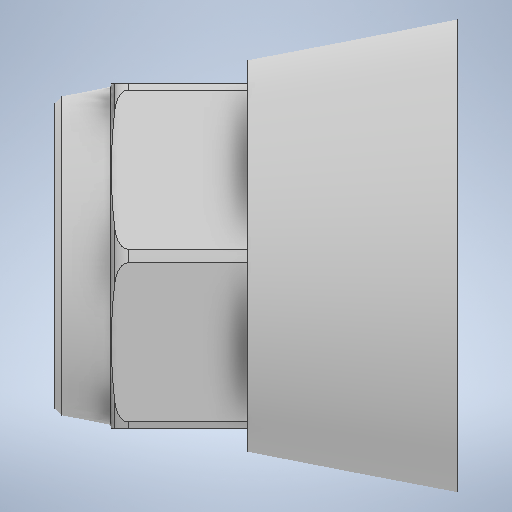
# Autodesk Inventor part: DT-HEX DWG_20251124
Saved by Autodesk Inventor 2025.3 (Build 293356000, 356)
## iProperties
Created: 2022-05-07
Part Number: DT-HEX DWG_20251124
Material: 일반
Document SubType Name: Modeling
Designer: shlee
Mass: 0.00932573 g
Surface Area: 0.529254 cm^2
Volume: 0.00932573 cm^3
Density: 1 g/cm^3
Appearance: 기본값
Author: shlee
Autodesk Inventor part; units mm, degrees
ref_plane "YZ Plane" through (0, 0, 0) normal (1, 0, 0) x (0, 1, 0)
ref_plane "XZ Plane" through (0, 0, 0) normal (0, 1, 0) x (-1, 0, 0)
ref_plane "XY Plane" through (0, 0, 0) normal (0, 0, 1) x (1, 0, 0)
sketch "스케치1" plane through (0, 0, 0) normal (1, 0, 0) x (0, 1, 0)
  line L0 (0, -0.2) -> (0, 12.7)
  line L1 (1.7039, -0.2) -> (1.41, 1.3119)
  line L2 (1.41, 1.3119) -> (1.41, 2.1718)
  line L3 (1.2179, 2.3) -> (1.1499, 2.65)
  line L4 (1.0999, 2.7) -> (0, 2.7)
  line L5 (0, 0) -> (1.665, 0) construction
  line L6 (1.1499, 2.65) -> (1.0999, 2.7)
  line L7 (1.7039, -0.2) -> (0, -0.2)
  arc A0 (1.41, 2.1718) -> (1.3359, 2.2684) centre (1.31, 2.1718) ccw
  line L8 (1.3359, 2.2684) -> (1.2179, 2.3)
  line L9 (0, 12.7) -> (7, 12.7)
  line L10 (7, 12.7) -> (7, 5.7)
  line L11 (2.5, 2.7) -> (1.0999, 2.7)
  line L12 (2.5, 2.7) -> (2.5, 5.7)
  line L13 (2.5, 5.7) -> (7, 5.7)
  line L14 (2.5, 2.7) -> (7, 2.7) construction
  line L15 (7, 2.7) -> (7, 5.7) construction
  line L16 (4, -1.973) -> (4, -0.9611) construction
  line L17 (4.2853, 6.1) -> (2.7419, 6.1) construction
  line L18 (7.3136, 3.3) -> (0.7648, 3.3) construction
  line L19 (2.5, 2.7) -> (2.5, 0) construction
  line L20 (7.2279, 2.7) -> (0.9279, 2.7) construction
  line L21 (0.9279, 2.7) -> (0.9279, 3.2) construction
  line L22 (0.9279, 3.2) -> (4.9116, 5.5) construction
  line L23 (4.9116, 5.5) -> (7.2279, 5.5) construction
  line L24 (7.2279, 5.5) -> (7.2279, 2.7) construction
  arc A1 (1.7039, -0.2) -> (1.9002, -0.3618) centre (1.9002, -0.1618) ccw
  line L25 (1.9002, -0.3618) -> (3.3915, -0.3618)
  arc A2 (1.753, -0.1905) -> (1.9002, -0.3118) centre (1.9002, -0.1618) ccw construction
  line L26 (1.9002, -0.3118) -> (3.3915, -0.3118) construction
  line L27 (1.753, -0.1905) -> (1.46, 1.3167) construction
  line L28 (1.46, 1.3167) -> (1.46, 2.1718) construction
  arc A3 (1.46, 2.1718) -> (1.3488, 2.3167) centre (1.31, 2.1718) ccw construction
  line L29 (1.3488, 2.3167) -> (1.261, 2.3402) construction
  line L30 (1.261, 2.3402) -> (1.1961, 2.6745) construction
  line L31 (1.1961, 2.6745) -> (1.1206, 2.75) construction
  line L32 (1.245, 2.4203) -> (1.245, 1.8412) construction
  line L33 (4.627, 2.8119) -> (1.627, 2.8119) construction
  line L34 (1.627, 2.8119) -> (1.627, 1.3119) construction
  line L35 (1.627, 1.3119) -> (4.627, 1.3119) construction
  line L36 (4.627, 1.3119) -> (4.627, 2.8119) construction
  line L37 (1.1206, 2.75) -> (1.0509, 2.75) construction
  line L38 (1.2605, 3.1402) -> (1.2605, 2.6402) construction
  line L39 (12.5384, 5.9) -> (9.4028, 5.9) construction
  line L40 (9.4028, 5.9) -> (9.4028, 3.9) construction
  line L41 (9.4028, 3.9) -> (12.5384, 3.9) construction
  line L42 (12.5384, 3.9) -> (12.5384, 5.9) construction
  point P0 (1.627, 2.0619)
  dimension "d10" = 3.33
  dimension "d26" = 0.05
  dimension "d27" = 135
  dimension "d423" = 1.3119
  dimension "d441" = 2.82
  dimension "d442" = 1.5119
  dimension "d448" = 0.1
  dimension "d453" = 0.2
  dimension "d459" = 2.9
  dimension "d460" = 75
  dimension "d461" = 0.4
  dimension "d462" = 0.8599
  dimension "d463" = 3.4078
  dimension "d464" = 2.3
  dimension "d465" = 11
  dimension "d466" = 14
  dimension "d468" = 5
  dimension "d470" = 10
  dimension "d471" = 8
  dimension "d472" = 0.9611
  dimension "d474" = 5.7
  dimension "d475" = 0.4
  dimension "d476" = 0.6
  dimension "d477" = 3
  dimension "d479" = 0.5
  dimension "d480" = 120
  dimension "d481" = 2.8
  dimension "d482" = 6.3
  dimension "d483" = 0.2
  dimension "d484" = 6.1
  dimension "d485" = 0.2
  dimension "d491" = 0.3118
  dimension "d492" = 0.05
  dimension "d497" = 0.15
  dimension "d498" = 2.92
  dimension "d499" = 1.5071
  dimension "d500" = 0.8551
  dimension "d501" = 2.6976
  dimension "d502" = 0.1449
  dimension "d503" = 0.15
  dimension "d504" = 2.49
  dimension "d505" = 0.0235
  dimension "d506" = 2.5221
  dimension "d507" = 3
  dimension "d508" = 1.5
  dimension "d510" = 3.8004
  dimension "d511" = 0.1214
  dimension "d512" = 3.5059
  dimension "d513" = 2.0619
  dimension "d514" = 0.3343
  dimension "d515" = 2.3921
  dimension "d516" = 0.05
  dimension "d517" = 0.0755
  dimension "d518" = 2.2412
  dimension "d519" = 0.5
  dimension "d520" = 0.3
  dimension "d521" = 2
  dimension "d522" = 0.2
  dimension "d523" = 3.9
  constraints: 87 end point, 12 horizontal, 8 point on circle, 7 perpendicular, 6 point on line, 6 vertical, 5 parallel, 5 tangent, 4 centre point, 2 collinear, 1 midpoint, 6 other
  measures "d10" diameter of L5.end L0
  measures "d26" horizontal distance of L3.end L4.start
  measures "d27" angle of L4 L6
  measures "d423" distance from line of L5 L1.end
  measures "d441" diameter of L2 L0
  measures "d442" distance from line of L7 L1.end
  measures "d448" radius of A0
  measures "d453" distance between parallel lines of L5 L7
  measures "d459" distance between parallel lines of L4 L7
  measures "d460" angle of L0 L8
  measures "d461" distance from line of L3.start L4
  measures "d462" distance of L1.end L2.end
  measures "d463" diameter of L1.start L0
  measures "d464" distance from line of L5 L3.start
  measures "d465" angle of L0 L1
  measures "d466" diameter of L10 L0
  measures "d468" diameter of L12 L0
  measures "d470" distance between parallel lines of L9 L14
  measures "d471" diameter of L16 L0
  measures "d472" distance from line of L5 L16.end
  measures "d474" distance between parallel lines of L13 L5
  measures "d475" distance between parallel lines of L13 L17
  measures "d476" distance between parallel lines of L4 L18
  measures "d477" distance between parallel lines of L13 L11
  measures "d479" distance of L20.end L21.end
  measures "d480" angle of L21 L22
  measures "d481" distance of L23.end L20.start
  measures "d482" distance between parallel lines of L21 L24
  measures "d483" distance between parallel lines of L13 L23
  measures "d484" distance between parallel lines of L17 L5
  measures "d485" radius of A1
  measures "d491" distance between parallel lines of L5 L26
  measures "d492" distance between parallel lines of L1 L27
  measures "d497" radius of A2
  measures "d498" diameter of L27.end L0
  measures "d499" vertical distance of L27.start L27.end
  measures "d500" distance of L27.end L28.end
  measures "d501" diameter of L29.start L0
  measures "d502" vertical distance of L28.end L29.start
  measures "d503" radius of A3
  measures "d504" diameter of L32 L0
  measures "d505" vertical distance of L29.start L29.end
  measures "d506" diameter of L29.end L0
  measures "d507" distance of L35.end L34.end
  measures "d508" distance of L34.end L33.end
  measures "d510" diameter of L26.start L0
  measures "d511" vertical distance of L26.start L27.start
  measures "d512" diameter of L27.start L0
  measures "d513" distance from line of point (1.627, 2.062) L5
  measures "d514" vertical distance of L29.end L30.end
  measures "d515" diameter of L30.end L0
  measures "d516" distance between parallel lines of L37 L20
  measures "d517" horizontal distance of L30.end L31.end
  measures "d518" diameter of L31.end L0
  measures "d519" distance of L38.start L38.end
  measures "d520" distance of L38.end L29.end
  measures "d521" distance of L39.end L40.end
  measures "d522" distance between parallel lines of L39 L13
  measures "d523" distance from line of L5.start L41
revolve "회전1" add sketch "스케치1" angle 360 about axis through (0, 0, -0.2) along (0, 0, 1) contours L0 L4 L6 L3 L8 A0 L2 L1 L7
sketch "스케치2" plane through (0, 0, 0) normal (1, 0, 0) x (0, 1, 0)
  line L0 (5.245, 1.3119) -> (1.245, 1.3119)
  line L1 (1.245, 1.3119) -> (1.245, 2.8119)
  line L2 (1.245, 2.8119) -> (5.245, 2.8119)
  line L3 (5.245, 2.8119) -> (5.245, 1.3119)
  line L4 (0, -1.7833) -> (0, 4.2492)
  line L5 (5.245, 2.0619) -> (1.245, 2.0619) construction
  line L6 (-1.0999, 2.7) -> (1.0999, 2.7) projected
  line L7 (-1.7039, -0.2) -> (1.7039, -0.2) projected
  point P0 (0, 0)
  dimension "d29" = 0
  dimension "d30" = 1.5
  dimension "d31" = 4
  dimension "d33" = 2.49
  dimension "d115" = -0.1119
  dimension "d233" = 1.3881
  dimension "d428" = 2.2619
  constraints: 12 end point, 3 horizontal, 3 vertical, 2 midpoint, 2 parallel, 1 perpendicular, 1 point on line, 8 other
  measures "d30" distance of L2.end L0.start
  measures "d31" distance of L2.start L2.end
  measures "d33" diameter of L1 L4
  measures "d115" distance between parallel lines of L2 L6
  measures "d233" distance between parallel lines of L6 L0
  measures "d428" distance between parallel lines of L7 L5
extrude "하부면취D1.5" cut sketch "스케치2" along normal mid plane 10
pattern_circular "원형 패턴1" count 6 over 360 about axis through (0, 0, -10) along (0, 0, 1) of "하부면취D1.5"
sketch "스케치24" plane through (0, 0, 0) normal (1, 0, 0) x (0, 1, 0)
  line L0 (0, -2.0054) -> (0, 3.6)
  line L1 (0, 3.6) -> (-1.0075, 2.9946)
  line L2 (-1.0075, 2.9946) -> (-1.0075, -2.0054)
  line L3 (-1.0075, -2.0054) -> (0, -2.0054)
  point P0 (0, 0)
  dimension "d454" = 59
  dimension "d455" = 2.015
  dimension "d456" = 5
  dimension "d457" = 3.6
  constraints: 8 end point, 2 vertical, 1 perpendicular, 1 point on line
  measures "d454" angle of L0 L1
  measures "d455" diameter of L2 L0
  measures "d456" distance of L1.end L2.end
  measures "d457" distance of L0.end point (0, 0)
revolve "회전7" cut sketch "스케치24" angle 360 about axis through (0, 0, -2.0054) along (0, 0, 1)
